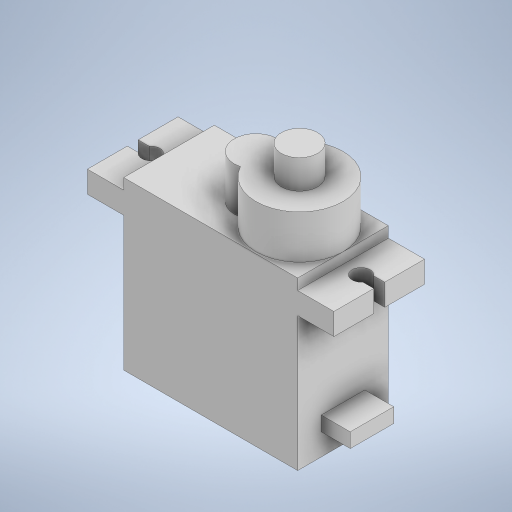
# Autodesk Inventor part: MG90_II
Saved by Autodesk Inventor 2023 (Build 270158000, 158)
## iProperties
Created: 2022-04-07
Part Number: MG90_II
Material: 一般
Document SubType Name: Modeling
Designer: device
Density: 1 g/cm^3
Appearance: 預設
Author: device
Autodesk Inventor part; units mm, degrees
ref_plane "YZ Plane" through (0, 0, 0) normal (1, 0, 0) x (0, 1, 0)
ref_plane "XZ Plane" through (0, 0, 0) normal (0, 1, 0) x (-1, 0, 0)
ref_plane "XY Plane" through (0, 0, 0) normal (0, 0, 1) x (1, 0, 0)
sketch "草圖1" plane through (0, 0, 0) normal (0, 0, 1) x (1, 0, 0)
  line L0 (-18, -14.5) -> (6, -14.5)
  line L1 (6, -14.5) -> (6, -33)
  line L2 (6, -33) -> (-18, -33)
  line L3 (-18, -33) -> (-18, -14.5)
  line L4 (-23, -11.5) -> (11, -11.5)
  line L5 (11, -11.5) -> (11, -14.5)
  line L6 (11, -14.5) -> (-23, -14.5)
  line L7 (-23, -14.5) -> (-23, -11.5)
  line L8 (6, -11.5) -> (-18, -11.5)
  line L9 (-18, -11.5) -> (-18, -10)
  line L10 (-18, -10) -> (6, -10)
  line L11 (6, -10) -> (6, -11.5)
  line L12 (6, -10) -> (-9, -10)
  line L13 (-9, -10) -> (-9, -4)
  line L14 (-9, -4) -> (6, -4)
  line L15 (6, -4) -> (6, -10)
  line L16 (2.5, -4) -> (-2.5, -4)
  line L17 (-2.5, -4) -> (-2.5, 0)
  line L18 (-2.5, 0) -> (2.5, 0)
  line L19 (2.5, 0) -> (2.5, -4)
  point P0 (0, 0)
  point P1 (-6, -14.5)
  point P2 (-6, -11.5)
  point P3 (0, -4)
  point P4 (-18, -11.5)
  point P5 (6, -14.5)
  point P6 (0, 0)
  dimension "d0" = 24
  dimension "d1" = 18.5
  dimension "d2" = 34
  dimension "d3" = 3
  dimension "d4" = 1.5
  dimension "d5" = 6
  dimension "d6" = 9
  dimension "d7" = 5
  dimension "d8" = 4
  dimension "d9" = 6
  constraints: 40 end point, 10 parallel, 6 midpoint, 5 horizontal, 5 perpendicular, 3 point on line, 2 collinear, 1 coincident
  measures "d0" distance of L1.end L2.end
  measures "d1" distance of L0.end L1.end
  measures "d2" distance of L5.end L6.end
  measures "d3" distance of L4.end L5.end
  measures "d4" distance of L10.end L8.start
  measures "d5" distance of L12.end L13.end
  measures "d6" horizontal distance of L9.end L13.end
  measures "d7" distance of L17.end L18.end
  measures "d8" distance of L16.end L17.end
  measures "d9" distance of L14.end point (0, -4)
extrude "擠出1" add sketch "草圖1" along normal mid plane 12.5 contours L6 L7 L4 L5 L0 | L0 L1 L2 L3 | L9 L10 L11 L4
sketch "草圖2" plane through (-18, -10, 6.25) normal (0, 1, 0) x (1, 0, 0)
  circle A0 centre (18, 6.25) radius 6
  circle A1 centre (12, 6.25) radius 3
  line L0 (0, 12.5) -> (0, 0) construction
  point P0 (9, 6.25)
  point P1 (0, 6.25)
  point P2 (12.75, 9.1547)
  point P3 (12.75, 3.3453)
  dimension "d13" = 12
  dimension "d14" = 9
  constraints: 1 coincident, 1 midpoint, 6 other
  measures "d14" distance of point (0, 6.25) point (9, 6.25)
extrude "擠出2" add sketch "草圖2" along normal blind 6
sketch "草圖3" plane through (-18, -4, 6.25) normal (0, 1, 0) x (1, 0, 0)
  circle A0 centre (18, 6.25) radius 2.5
  dimension "d17" = 5
  constraints: 1 centre point, 1 coincident
  measures "d17" diameter of A0
extrude "擠出3" add sketch "草圖3" along normal blind 4
sketch "草圖4" plane through (-23, -11.5, 6.25) normal (0, 1, 0) x (1, 0, 0)
  line L0 (0, 12.5) -> (0, 0) construction
  line L1 (5, 0) -> (0, 0) construction
  line L2 (5, 12.5) -> (5, 0) construction
  line L3 (0, 12.5) -> (5, 12.5) construction
  line L4 (0, 6.25) -> (5, 6.25) construction
  circle A0 centre (2.5, 6.25) radius 1.25
  line L5 (0, 12.5) -> (0, 0) projected
  line L6 (0, 7) -> (1.5, 7)
  line L7 (1.5, 7) -> (1.5, 5.5)
  line L8 (1.5, 5.5) -> (0, 5.5)
  line L9 (0, 5.5) -> (0, 7)
  line L10 (0, 9.2582) -> (34, 9.2582) construction
  line L11 (34, 12.5) -> (34, 0) projected
  line L12 (17, 9.2582) -> (17, 6.5712) construction
  circle A1 centre (31.5, 6.25) radius 1.25
  line L13 (34, 7) -> (32.5, 7)
  line L14 (32.5, 7) -> (32.5, 5.5)
  line L15 (32.5, 5.5) -> (34, 5.5)
  line L16 (34, 5.5) -> (34, 7)
  point P0 (23, 6.25)
  point P1 (0, 5.5)
  point P2 (1.5, 7)
  point P3 (34, 6.25)
  dimension "d20" = 2.5
  dimension "d21" = 1.5
  dimension "d22" = 14.5
  constraints: 22 end point, 6 symmetric about line, 4 midpoint, 3 point on line, 2 horizontal, 2 parallel, 2 vertical, 1 perpendicular, 7 other
  measures "d21" distance of L6.end L7.end
  measures "d22" distance from line of L12 point (2.5, 6.25)
extrude "擠出4" cut sketch "草圖4" against normal up to surface (3 mm away)
sketch "草圖5" plane through (6, -33, 6.25) normal (1, 0, 0) x (0, 0, -1)
  line L0 (12.5, 18.5) -> (0, 18.5) construction
  line L1 (0, 0) -> (0, 18.5) construction
  line L2 (12.5, 0) -> (0, 0) construction
  line L3 (12.5, 18.5) -> (12.5, 0) construction
  line L4 (0, 18.5) -> (0, 0) construction
  line L5 (0, 5) -> (3.25, 5) construction
  line L6 (3.25, 5) -> (9.25, 5)
  line L7 (9.25, 5) -> (9.25, 3)
  line L8 (9.25, 3) -> (3.25, 3)
  line L9 (3.25, 3) -> (3.25, 5)
  line L10 (3.25, 5) -> (9.25, 5)
  line L11 (9.25, 5) -> (12.5, 5) construction
  point P0 (6.25, 33)
  dimension "d25" = 6
  dimension "d26" = 13.5
  dimension "d27" = 3
  constraints: 14 end point, 4 perpendicular, 2 parallel, 2 point on line, 1 collinear, 1 horizontal
  measures "d25" distance of L5.end L6.end
  measures "d26" distance between parallel lines of L0 L6
  measures "d27" distance between parallel lines of L2 L8
extrude "擠出5" add sketch "草圖5" along normal blind 4
